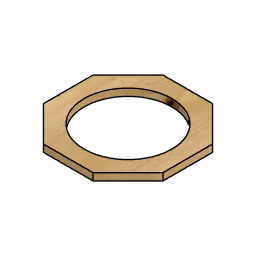
digitalclock_frame (Autodesk Fusion 360 design; units mm, degrees)
Autodesk Fusion 360 part; units mm, degrees
sketch "Skizze1" plane through (0, 0, 0) normal (0, 0, 1) x (1, 0, 0)
  line L0 (-87.8679, 0) -> (-212.132, 0)
  line L1 (-300, -87.868) -> (-300, -212.132)
  line L2 (-212.132, -300) -> (-87.8679, -300)
  line L3 (0, -212.1321) -> (0, -87.8679)
  line L4 (0, -87.8679) -> (-87.8679, 0)
  line L5 (-212.132, 0) -> (-300, -87.868)
  line L6 (-300, -212.132) -> (-212.132, -300)
  line L7 (-87.8679, -300) -> (0, -212.1321)
  dimension "d3" = 45
  dimension "d4" = 45
  dimension "d5" = 300
  dimension "d6" = 300
  dimension "d9" = 87.8679
  dimension "d10" = 87.8679
  dimension "d11" = 300
  dimension "d12" = 300
  constraint horizontal L0
  constraint vertical L1
  constraint horizontal L2
  constraint vertical L3
  constraint parallel L4 L6
  constraint parallel L5 L7
  constraint coincident origin L0
  constraint coincident origin L3
  measures "d3" angle of L3 L7
  measures "d4" angle of L3 L4
  measures "d5" distance of L5 L7
  measures "d6" distance of L4 L6
  measures "d9" distance of origin L3.end
  measures "d10" vertical distance of L2.end L3.start
  measures "d11" distance of L1 L3
  measures "d12" distance of L0 L2
extrude "Extrusion1" add sketch "Skizze1" along normal blind 18
sketch "Skizze2" plane through (0, 0, 18) normal (0, 0, 1) x (-1, 0, 0)
  line L0 (87.8679, 300) -> (0, 212.1321)
  line L1 (0, 212.1321) -> (0, 87.8679)
  line L2 (0, 87.8679) -> (87.8679, 0)
  line L3 (87.8679, 0) -> (212.132, 0)
  line L4 (212.132, 0) -> (300, 87.868)
  line L5 (300, 87.868) -> (300, 212.132)
  line L6 (300, 212.132) -> (212.132, 300)
  line L7 (212.132, 300) -> (87.8679, 300)
  circle A0 centre (150, 150) radius 110
  dimension "d15" = 150
  dimension "d16" = 150
  dimension "d17" = 220
  measures "d15" horizontal distance of origin A0.centre
  measures "d16" vertical distance of origin A0.centre
  measures "d17" diameter of A0
extrude "Extrusion2" cut sketch "Skizze2" against normal blind 18 contours A0
sketch "Skizze3" plane through (0, 0, 0) normal (0, 0, -1) x (1, 0, 0)
  circle A0 centre (-150, 150) radius 110
  line L0 (0, 212.1321) -> (-87.8679, 300)
  line L1 (-87.8679, 300) -> (-212.132, 300)
  line L2 (-212.132, 300) -> (-300, 212.132)
  line L3 (-300, 212.132) -> (-300, 87.868)
  line L4 (-300, 87.868) -> (-212.132, 0)
  line L5 (-212.132, 0) -> (-87.8679, 0)
  line L6 (-87.8679, 0) -> (0, 87.8679)
  line L7 (0, 87.8679) -> (0, 212.1321)
  line L8 (-65.2405, 90.5097) -> (-51.0983, 76.3675)
  line L9 (-51.0983, 76.3675) -> (-79.3826, 48.0833)
  line L10 (-79.3826, 48.0833) -> (-93.5248, 62.2254)
  line L11 (-93.5248, 62.2254) -> (-65.2405, 90.5097)
  dimension "d20" = 28
  dimension "d21" = 40
  dimension "d22" = 40
  dimension "d23" = 20
  constraint perpendicular L8 L9
  constraint perpendicular L9 L10
  constraint parallel L6 L9
  constraint parallel L9 L11
  measures "d20" distance of L6 L9
  measures "d21" distance of L8 L10
  measures "d22" distance of L5.end L10
  measures "d23" distance of L9 L11
extrude "Extrusion3" cut sketch "Skizze3" against normal blind 10 contours A0 L8 L9 L10
sketch "Skizze4" plane through (0, 0, 0) normal (0, 1, 0) x (-1, 0, 0)
  line L0 (87.8679, 0) -> (212.132, 0)
  line L1 (212.132, 0) -> (212.132, 18)
  line L2 (212.132, 18) -> (87.8679, 18)
  line L3 (87.8679, 18) -> (87.8679, 0)
  line L4 (144.8679, 6.5) -> (154.8679, 6.5)
  arc A0 (154.8679, 6.5) -> (154.8679, 11.5) centre (154.8679, 9) ccw
  line L5 (154.8679, 11.5) -> (144.8679, 11.5)
  arc A1 (144.8679, 11.5) -> (144.8679, 6.5) centre (144.8679, 9) ccw
  dimension "d26" = 5
  dimension "d27" = 10
  dimension "d28" = 9
  dimension "d30" = 57
  constraint horizontal L4
  constraint tangent L4 A0
  constraint tangent A0 L5
  constraint parallel L4 L5
  constraint tangent L5 A1
  constraint tangent L4 A1
  measures "d26" distance of L4 L5
  measures "d27" distance of A0.centre A1.centre
  measures "d28" distance of L2 A1.centre
  measures "d30" horizontal distance of L0.start A1.centre
extrude "Extrusion4" cut sketch "Skizze4" against normal blind 20 contours L4 A0 L5 A1
sketch "Skizze5" plane through (0, -20, 0) normal (0, 1, 0) x (-1, 0, 0)
  arc A0 (144.8679, 11.5) -> (144.8679, 6.5) centre (144.8679, 9) ccw
  line L0 (144.8679, 6.5) -> (154.8679, 6.5)
  arc A1 (154.8679, 6.5) -> (154.8679, 11.5) centre (154.8679, 9) ccw
  line L1 (154.8679, 11.5) -> (144.8679, 11.5)
  circle A2 centre (149.8679, 9) radius 2.5
  dimension "d33" = 5
  dimension "d34" = 5
  dimension "d35" = 2.5
  measures "d33" diameter of A2
  measures "d34" distance of A1.centre A2.centre
  measures "d35" distance of L0 A2.centre
extrude "Extrusion5" cut sketch "Skizze5" against normal blind 40 contours A2
equation "d30 = ( 124 / 2 ) * 1 mm - 5 mm"
